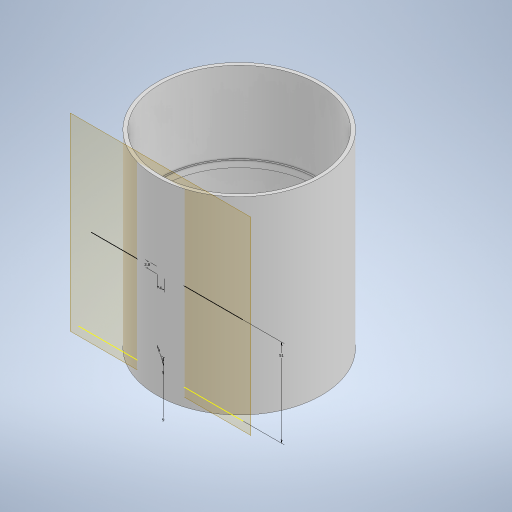
# Autodesk Inventor part: 탄두옆면1
Saved by Autodesk Inventor 2023 (Build 270158000, 158)
## iProperties
Created: 2023-10-31
Part Number: 탄두옆면1
Material: 일반
Document SubType Name: Modeling
Designer: rlatk
Density: 1 g/cm^3
Appearance: 기본값
Author: rlatk
Autodesk Inventor part; units mm, degrees
ref_plane "YZ Plane" through (0, 0, 0) normal (1, 0, 0) x (0, 1, 0)
ref_plane "XZ Plane" through (0, 0, 0) normal (0, 1, 0) x (-1, 0, 0)
sketch "스케치1" plane through (0, 0, 0) normal (0, 1, 0) x (-1, 0, 0)
  circle A0 centre (0, 0) radius 45.85
  circle A1 centre (0, 0) radius 47.85
  dimension "d0" = 91.7
  dimension "d1" = 2
  constraints: 2 centre point, 1 coincident
  measures "d0" diameter of A0
  measures "d1" radial gap between concentric circles of A0 A1
extrude "돌출1" add sketch "스케치1" along normal blind 100
ref_plane "작업 평면1" through (0, 0, 45.75) normal (0, 0, 1) x (1, 0, 0)
sketch "스케치2" plane through (0, 0, 45.75) normal (0, 0, 1) x (1, 0, 0)
  circle A0 centre (0, 9) radius 4.5
  line L0 (47.85, 0) -> (-47.85, 0) projected
  line L1 (-40.336, 51) -> (47.75, 51)
  line L2 (2, 52.9) -> (-2, 52.9)
  line L3 (-2, 52.9) -> (-2, 49.1)
  line L4 (-2, 49.1) -> (2, 49.1)
  line L5 (2, 49.1) -> (2, 52.9)
  line L6 (2, 52.9) -> (-2, 49.1) construction
  line L7 (-2, 52.9) -> (2, 49.1) construction
  point P0 (0, 0)
  point P1 (0, 51)
  dimension "d5" = 9
  dimension "d6" = 9
  dimension "d10" = 51
  dimension "d11" = 4
  dimension "d12" = 3.8
  constraints: 14 end point, 2 horizontal, 2 midpoint, 2 parallel, 1 centre point, 1 perpendicular, 1 point on line
  measures "d5" diameter of A0
  measures "d6" distance from line of L0 A0.centre
  measures "d10" distance between parallel lines of L1 L0
  measures "d11" distance of L4.end L3.end
  measures "d12" distance of L3.end L2.end
extrude "돌출2" add sketch "스케치2" against normal blind 10 contours A0
fillet "모깎기1" radius 2 1 edges at (-4.5, 9, 35.75)
sketch "스케치3" plane through (0, 0, 0) normal (1, 0, 0) x (0, 1, 0)
  line L0 (100, 45.85) -> (0, 45.85) projected
  line L1 (-20, 0) -> (120, 0) projected
  line L2 (100, 45.85) -> (0, 45.85) projected
  line L3 (52.9, 45.85) -> (49.1, 45.85)
  line L4 (49.1, 45.85) -> (49.1, 44.85)
  line L5 (49.1, 44.85) -> (52.9, 44.85)
  line L6 (52.9, 44.85) -> (52.9, 45.85)
  point P0 (0, 0)
  point P1 (49.1, 45.75)
  point P2 (49.1, 45.75)
  point P3 (49.1, 45.75)
  point P4 (52.9, 45.75)
  point P5 (52.9, 45.75)
  point P6 (52.9, 45.75)
  dimension "d17" = 1
  constraints: 8 end point, 2 parallel, 1 horizontal, 1 perpendicular, 1 point on line, 1 other
  measures "d17" distance of L4.end L3.end
sketch "스케치4" plane through (0, 0, 0) normal (0, -1, 0) x (1, 0, 0)
  point P0 (0, 0)
revolve "회전2" add sketch "스케치3" angle 360 about axis through (0, -10, 0) along (0, 1, 0)
sketch "스케치5" plane through (0, 0, 0) normal (0, -1, 0) x (1, 0, 0)
  circle A0 centre (0, 0) radius 45.85 projected
  circle A1 centre (0, 0) radius 47.85 projected
  circle A2 centre (0, 0) radius 45.85
  circle A3 centre (0, 0) radius 47.85
  constraints: 2 centre point, 2 coincident, 2 concentric
extrude "돌출4" add sketch "스케치5" along normal blind 10
sketch "스케치6" plane through (0, 0, 45.75) normal (0, 0, 1) x (1, 0, 0)
  point P0 (0, 0)
sketch "스케치7" plane through (0, 0, 0) normal (1, 0, 0) x (0, 1, 0)
  line L0 (49.1, 45.85) -> (-10, 45.85) projected
  line L1 (-9, 45.85) -> (-7, 45.85)
  line L2 (-7, 45.85) -> (-7, 43.85)
  line L3 (-7, 43.85) -> (-9, 43.85)
  line L4 (-9, 43.85) -> (-9, 45.85)
  line L5 (-9, 45.85) -> (-8.5, 43.85)
  line L6 (-7, 45.85) -> (-7.5, 43.85)
  point P0 (0, 0)
  dimension "d21" = 2
  dimension "d22" = 2
  dimension "d23" = 1
  dimension "d24" = 0.5
  dimension "d25" = 0.5
  constraints: 12 end point, 3 point on line, 2 parallel, 1 horizontal, 1 perpendicular
  measures "d21" distance of L2.end L3.end
  measures "d22" distance of L1.end L2.end
  measures "d23" distance of L1.start L0.end
  measures "d24" distance of L5.end L3.end
  measures "d25" distance of L2.end L6.end
coil "코일1" sketch "스케치7" operation add axis through (0, -10, 0) along (0, 1, 0) pitch 4 turns 2 hand right contours L6 L3 L5 L0
